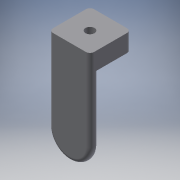
# Autodesk Inventor part: NASA-20-ARM-HG-01
Saved by Autodesk Inventor 2019 (Build 230136000, 136)
## iProperties
Created: 2019-09-09
Part Number: NASA-20-ARM-HG-01
Material: Generic
Document SubType Name: Modeling
Designer: Rick Szalay
Density: 1 g/cm^3
Appearance: Default
Author: Rick Szalay
Autodesk Inventor part; units mm, degrees
ref_plane "YZ Plane" through (0, 0, 0) normal (1, 0, 0) x (0, 1, 0)
ref_plane "XZ Plane" through (0, 0, 0) normal (0, 1, 0) x (-1, 0, 0)
ref_plane "XY Plane" through (0, 0, 0) normal (0, 0, 1) x (1, 0, 0)
sketch "Sketch1" plane through (0, 0, 0) normal (0, 0, 1) x (1, 0, 0)
  arc A0 (-15, 0) -> (15, 0) centre (0, 0) ccw
  line L0 (-15, 60) -> (15, 60)
  line L1 (15, 60) -> (15, 0)
  line L2 (-15, 0) -> (-15, 60)
  dimension "d0" = 30
  dimension "d1" = 60
  constraints: 6 end point, 2 point on circle, 2 tangent, 1 centre point, 1 coincident, 1 horizontal, 1 parallel, 1 perpendicular
  measures "d0" diameter of A0
  measures "d1" distance from line of point (0, 0) L0
extrude "Extrusion1" add sketch "Sketch1" along normal mid plane 30
sketch "Sketch2" plane through (0, 0, -15) normal (0, 0, -1) x (-1, 0, 0)
  arc A0 (-15, 0) -> (15, 0) centre (0, 0) ccw
  line L0 (15, 0) -> (15, 47.3)
  line L1 (15, 47.3) -> (-15, 47.3)
  line L2 (-15, 47.3) -> (-15, 0)
  line L3 (15, 0) -> (15, 60) projected
  line L4 (-15, 60) -> (-15, 0) projected
  line L5 (15, 60) -> (-15, 60) projected
  dimension "d4" = 12.7
  constraints: 6 end point, 2 collinear, 2 point on circle, 2 tangent, 1 centre point, 1 coincident, 1 parallel, 1 perpendicular, 1 vertical
  measures "d4" distance between parallel lines of L1 L5
extrude "Extrusion2" cut sketch "Sketch2" against normal blind 23.65 contours L2 L1 L0 A0
fillet "Fillet1" radius 3 11 edges at (-15, 53.65, -15) (15, 53.65, -15) (0, -15, 15) (15, 30, 15) (-15, 30, 15) (0, -15, 8.65) (15, 23.65, 8.65) (-15, 23.65, 8.65) (-15, 47.3, -3.175) (0, 47.3, -15) (15, 47.3, -3.175)
sketch "Sketch3" plane through (-12, 47.3, -15) normal (0, -1, 0) x (1, 0, 0)
  point P0 (12, 15)
  point P1 (12, 15)
  constraints: 1 coincident
hole "Hole1" at (0, 47.3, 0) direction (0, 1, 0) diameter 6.604 end through all counterbore diameter 16.51 counterbore depth 4.8006 clearance for "Hex Head Cap Screw DIN EN 24017" size "M6" standard "DIN"
sketch "Sketch4" plane through (0, 0, 15) normal (0, 0, 1) x (1, 0, 0)
  point P0 (0, 0)
  point P1 (0, 0)
  constraints: 1 coincident
hole "Hole2" at (0, 0, 15) direction (0, 0, -1) diameter 6 end through all
body "Solid1"
